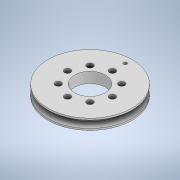
# Autodesk Inventor part: Pully_r12
Saved by Autodesk Inventor 2021 (Build 250183000, 183)
## iProperties
Created: 2022-09-22
Part Number: Pully_r12
Material: Generic
Document SubType Name: Modeling
Designer: ereg140
Density: 1 g/cm^3
Appearance: Default
Author: ereg140
Autodesk Inventor part; units mm, degrees
ref_plane "YZ Plane" through (0, 0, 0) normal (1, 0, 0) x (0, 1, 0)
ref_plane "XZ Plane" through (0, 0, 0) normal (0, 1, 0) x (-1, 0, 0)
ref_plane "XY Plane" through (0, 0, 0) normal (0, 0, 1) x (1, 0, 0)
sketch "Sketch1" plane through (0, 0, 0) normal (0, 1, 0) x (-1, 0, 0)
  circle A0 centre (0, 0) radius 15
  dimension "d0" = 30
  constraints: 1 centre point, 1 coincident
  measures "d0" diameter of A0
extrude "Extrusion1" add sketch "Sketch1" along normal blind 3.8
sketch "Sketch2" plane through (0, 3.8, 0) normal (0, 1, 0) x (1, 0, 0)
  circle A0 centre (0, 0) radius 8 construction
  circle A1 centre (-8, 0) radius 1.1
  circle A2 centre (-5.6569, -5.6569) radius 1.1
  circle A3 centre (0, -8) radius 1.1
  circle A4 centre (5.6569, -5.6569) radius 1.1
  circle A5 centre (8, 0) radius 1.1
  circle A6 centre (5.6569, 5.6569) radius 1.1
  circle A7 centre (0, 8) radius 1.1
  circle A8 centre (-5.6569, 5.6569) radius 1.1
  circle A9 centre (0, 0) radius 5.5
  dimension "d3" = 16
  dimension "d4" = 2.2
  dimension "d7" = 360
  dimension "d9" = 11
  constraints: 9 centre point, 2 coincident, 2 horizontal alignment, 19 other
  measures "d4" diameter of A1
  measures "d9" diameter of A9
extrude "Extrusion2" cut sketch "Sketch2" against normal through all
sketch "Sketch3" plane through (0, 0, 0) normal (1, 0, 0) x (0, 1, 0)
  point P0 (0, 0)
sketch "Sketch4" plane through (0, 0, 0) normal (1, 0, 0) x (0, 1, 0)
  line L0 (3.8, 5.5) -> (0, 5.5) construction
  line L1 (0, 5.5) -> (0, 6.9) construction
  line L2 (0, 6.9) -> (3.8, 6.9) construction
  line L3 (3.8, 6.9) -> (3.8, 5.5) construction
  line L4 (0, -5.5) -> (3.8, -5.5) construction
  line L5 (3.8, -5.5) -> (3.8, -6.9) construction
  line L6 (3.8, -6.9) -> (0, -6.9) construction
  line L7 (0, -6.9) -> (0, -5.5) construction
  line L8 (0, 15) -> (3.8, 15) construction
  line L9 (3.8, 15) -> (3.8, 9.1) construction
  line L10 (3.8, 9.1) -> (0, 9.1) construction
  line L11 (0, 9.1) -> (0, 15) construction
  line L12 (3.8, -15) -> (0, -15) construction
  line L13 (0, -15) -> (0, -9.1) construction
  line L14 (0, -9.1) -> (3.8, -9.1) construction
  line L15 (3.8, -9.1) -> (3.8, -15) construction
  line L16 (0.6, -15) -> (3.2, -15)
  line L17 (3.2, -15) -> (3.2, -12)
  line L18 (3.2, -12) -> (0.6, -12)
  line L19 (0.6, -12) -> (0.6, -15)
  line L20 (-0.76, 0) -> (4.56, 0) projected
  point P0 (0, 0)
  point P1 (1.9, -15)
  dimension "d12" = 0.6
  dimension "d15" = 12
  constraints: 8 end point, 2 midpoint, 2 parallel, 1 horizontal, 1 perpendicular
  measures "d12" distance between parallel lines of L13 L19
  measures "d15" distance from line of point (0, 0) L18
revolve "Revolution1" cut sketch "Sketch4" angle 360 about axis through (0, -10, 0) along (0, 1, 0)
sketch "Sketch5" plane through (0, 3.2, 0) normal (0, -1, 0) x (1, 0, 0)
  circle A0 centre (0, -12.6) radius 0.6
  circle A1 centre (0, 0) radius 12 construction
  circle A2 centre (0, 0) radius 15 construction
  circle A3 centre (-8, 0) radius 1.1 construction
  circle A4 centre (8, 0) radius 1.1 construction
  circle A5 centre (5.6569, 5.6569) radius 1.1 construction
  circle A6 centre (-5.6569, -5.6569) radius 1.1 construction
  circle A7 centre (-5.6569, 5.6569) radius 1.1 construction
  circle A8 centre (5.6569, -5.6569) radius 1.1 construction
  circle A9 centre (0, 8) radius 1.1 construction
  circle A10 centre (0, -8) radius 1.1 construction
  circle A11 centre (0, 0) radius 5.5 construction
  dimension "d17" = 1.2
  constraints: 1 centre point, 1 tangent, 1 vertical alignment
  measures "d17" diameter of A0
extrude "Extrusion3" cut sketch "Sketch5" against normal up to surface (0.6 mm away)
body "Solid1"
